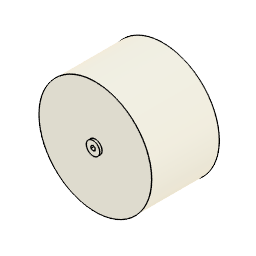
Rear Drivetrain (Autodesk Fusion 360 archive; units mm, degrees)
design "Rear Wheel"
Autodesk Fusion 360 part; units mm, degrees
sketch "スケッチ1" plane through (0, 0, 0) normal (0, 1, 0) x (1, 0, 0)
  circle A0 centre (0, 0) radius 25
  dimension "d1" = 50
  constraint coincident A0.centre origin
  measures "d1" diameter of A0
extrude "押し出し1" add sketch "スケッチ1" along normal blind 30
sketch "スケッチ2" plane through (0, 0, 0) normal (0, -1, 0) x (1, 0, 0)
  circle A0 centre (0, 0) radius 25
  circle A1 centre (0, 0) radius 3
  line L0 (0, 1.05) -> (-0.9093, 0.525)
  line L1 (-0.9093, 0.525) -> (-0.9093, -0.525)
  line L2 (-0.9093, -0.525) -> (0, -1.05)
  line L3 (0, -1.05) -> (0.9093, -0.525)
  line L4 (0.9093, -0.525) -> (0.9093, 0.525)
  line L5 (0.9093, 0.525) -> (0, 1.05)
  dimension "d4" = 6
  dimension "d5" = 2.1
  constraint coincident A0.centre A1.centre
  measures "d4" diameter of A1
  measures "d5" distance of L0.start L2.end
extrude "押し出し2" add sketch "スケッチ2" along normal blind 1 contours A1
extrude "押し出し3" cut 1 faces at (0, 0, 0.35) along direction (0, 1, 0) blind 4

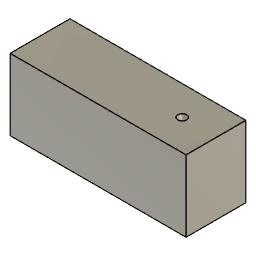
design "モーター"
Autodesk Fusion 360 part; units mm, degrees
sketch "スケッチ1" plane through (0, 0, 0) normal (0, 0, 1) x (1, 0, 0)
  line L0 (0, 0) -> (69, 0)
  line L1 (69, 0) -> (69, 23.5)
  line L2 (69, 23.5) -> (0, 23.5)
  line L3 (0, 23.5) -> (0, 0)
  circle A0 centre (55.5, 12) radius 1.75
  dimension "d1" = 12
  dimension "d2" = 3.5
  dimension "d3" = 23.5
  dimension "d4" = 69
  dimension "d5" = 13.5
  constraint horizontal L0
  constraint vertical L1
  constraint horizontal L2
  constraint vertical L3
  constraint coincident L0.start L3.end
  measures "d1" distance of L0 A0.centre
  measures "d2" diameter of A0
  measures "d3" distance of L0.end L1.end
  measures "d4" distance of L1.end L2.end
  measures "d5" distance of L1 A0.centre
extrude "押し出し1" add sketch "スケッチ1" along normal blind 28

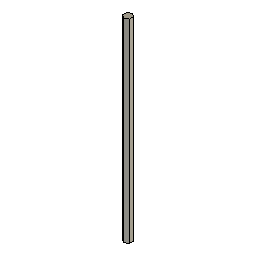
design "リアシャフト"
Autodesk Fusion 360 part; units mm, degrees
sketch "スケッチ1" plane through (0, 0, 0) normal (0, 0, 1) x (1, 0, 0)
  line L0 (1.299, -0.75) -> (1.299, 0.75)
  line L1 (1.299, 0.75) -> (0, 1.5)
  line L2 (0, 1.5) -> (-1.299, 0.75)
  line L3 (-1.299, 0.75) -> (-1.299, -0.75)
  line L4 (-1.299, -0.75) -> (0, -1.5)
  line L5 (0, -1.5) -> (1.299, -0.75)
  dimension "d1" = 1.5
  measures "d1" distance of L0.start origin
extrude "押し出し1" add sketch "スケッチ1" along normal blind 70
equation "d2 = 28 mm + ( 21 * 2 ) * 1 mm"
